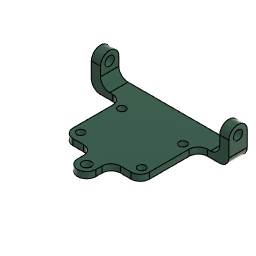
Car_Frame (Autodesk Fusion 360 archive; units mm, degrees)
design "Camera Mount v2"
Autodesk Fusion 360 part; units mm, degrees
sketch "Sketch1" plane through (0, 0, 0) normal (0, 0, 1) x (1, 0, 0)
  line L0 (12.5, 12.5) -> (-12.5, 12.5)
  line L1 (-12.5, 12.5) -> (-12.5, -12.5)
  line L2 (-12.5, -12.5) -> (12.5, -12.5)
  line L3 (12.5, -12.5) -> (12.5, 12.5)
  line L4 (12.5, 12.5) -> (-12.5, -12.5) construction
  line L5 (-12.5, 12.5) -> (12.5, -12.5) construction
  line L6 (10, 4) -> (-10, 4) construction
  line L7 (-10, 4) -> (-10, -9.5) construction
  line L8 (-10, -9.5) -> (10, -9.5) construction
  line L9 (10, -9.5) -> (10, 4) construction
  line L10 (10, 4) -> (-10, -9.5) construction
  line L11 (-10, 4) -> (10, -9.5) construction
  line L12 (0, 0) -> (0, -2.75) construction
  circle A0 centre (-10, -9.5) radius 1.25
  circle A1 centre (-10, 4) radius 1.25
  circle A2 centre (10, 4) radius 1.25
  circle A3 centre (10, -9.5) radius 1.25
  line L13 (-22.5, 12.5) -> (22.5, 12.5)
  line L14 (22.5, 12.5) -> (22.5, 6.5)
  line L15 (22.5, 6.5) -> (-22.5, 6.5)
  line L16 (-22.5, 6.5) -> (-22.5, 12.5)
  line L17 (-12.5, 0) -> (12.5, 0) construction
  line L18 (-22.5, -6.5) -> (-22.5, -12.5) construction
  line L19 (-22.5, -12.5) -> (22.5, -12.5) construction
  line L20 (22.5, -6.5) -> (-22.5, -6.5) construction
  line L21 (22.5, -12.5) -> (22.5, -6.5) construction
  circle A4 centre (0, -17.5) radius 1.5
  line L22 (-3, -17.5) -> (-3, -12.5)
  line L23 (3, -17.5) -> (3, -12.5)
  arc A5 (-3, -17.5) -> (3, -17.5) centre (0, -17.5) ccw
  point P0 (0, -2.75)
  dimension "d1" = 25
  dimension "d2" = 25
  dimension "d3" = 13.5
  dimension "d4" = 20
  dimension "d5" = 3
  dimension "d6" = 2.5
  dimension "d7" = 2.5
  dimension "d8" = 2.5
  dimension "d9" = 2.5
  dimension "d12" = 45
  dimension "d13" = 6
  dimension "d24" = 3
  dimension "d25" = 6
  dimension "d26" = 5
  constraint horizontal L0
  constraint perpendicular L0 L1
  constraint parallel L0 L2
  constraint parallel L1 L3
  constraint coincident L4 L12.start
  constraint coincident L5 L12.start
  constraint coincident L12.start origin
  constraint horizontal L6
  constraint perpendicular L6 L7
  constraint parallel L6 L8
  constraint parallel L7 L9
  constraint coincident L10 P0
  constraint coincident L11 P0
  constraint coincident P0 L12.end
  constraint vertical L12
  constraint coincident L7.end L8.start
  constraint coincident L6.end L7.start
  constraint coincident L6.start L9.end
  constraint coincident L8.end L9.start
  constraint horizontal L13
  constraint vertical L14
  constraint horizontal L15
  constraint vertical L16
  constraint collinear L0 L13
  constraint symmetric L12 L14 L16
  constraint midpoint L1 L17.start
  constraint midpoint L3 L17.end
  constraint symmetric L13.start L17 L18.end
  constraint symmetric L13.end L17 L19.end
  constraint symmetric L14.end L17 L20.start
  constraint symmetric L15.end L17 L18.start
  constraint concentric A4 A5
  constraint coincident L2 L22.end
  constraint coincident L2 L23.end
  constraint vertical L23
  constraint vertical L22
  constraint tangent L22 A5
  constraint tangent L23 A5
  constraint coincident L12 A4.centre
  measures "d1" distance of L1.end L2.end
  measures "d2" distance of L0.end L1.end
  measures "d3" distance of L6.end L7.end
  measures "d4" distance of L6.start L6.end
  measures "d5" distance of L2 L8
  measures "d6" diameter of A0
  measures "d7" diameter of A1
  measures "d8" diameter of A2
  measures "d9" diameter of A3
  measures "d12" distance of L13.start L13.end
  measures "d13" distance of L13.end L14.end
  measures "d24" diameter of A4
  measures "d25" diameter of A5
  measures "d26" distance of L2 A4.centre
extrude "Extrude1" add sketch "Sketch1" along normal blind 2
sketch "Sketch2" plane through (0, 0, 0) normal (1, 0, 0) x (0, 1, 0)
  line L0 (12.5, 0) -> (6.5, 0)
  line L1 (6.5, 0) -> (6.5, 2)
  line L2 (6.5, 2) -> (12.5, 2)
  line L3 (12.5, 2) -> (12.5, 0)
  line L4 (9.5, 2) -> (9.5, 8) construction
  circle A0 centre (9.5, 8) radius 1.5
  circle A1 centre (9.5, 8) radius 3
  line L5 (12.5, 2) -> (12.5, 8)
  line L6 (6.5, 2) -> (6.5, 8)
  dimension "d15" = 3
  dimension "d16" = 6
  dimension "d17" = 6
  constraint midpoint L2 L4.start
  constraint perpendicular L2 L4
  constraint coincident L4.end A0.centre
  constraint concentric A0 A1
  constraint coincident L2.end L3.start
  constraint coincident A1 L5.end
  constraint tangent A1 L5
  constraint coincident L1.end L2.start
  constraint coincident A1 L6.end
  constraint tangent A1 L6
  constraint vertical L6
  constraint vertical L5
  measures "d15" diameter of A0
  measures "d16" diameter of A1
  measures "d17" distance of L4.start L4.end
extrude "Extrude2" add sketch "Sketch2" along normal blind 3 from surface at -22.5 contours L2 A1 L5 L6 | A1
extrude "Extrude3" add sketch "Sketch2" against normal blind 3 from surface at 22.5 contours L2 A1 L5 L6 | A1
fillet "Fillet1" radius 3 10 edges at (12.5, 6.5, 1) (-12.5, 6.5, 1) (-12.5, -12.5, 1) (12.5, -12.5, 1) (-22.5, 9.5, 0) (22.5, 9.5, 0) (-19.5, 9.5, 2) (19.5, 9.5, 2) (3, -12.5, 1) (-3, -12.5, 1)

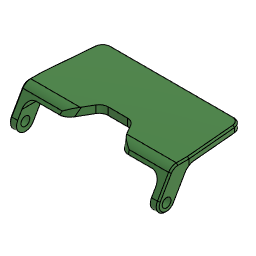
design "Camera Protector"
Autodesk Fusion 360 part; units mm, degrees
sketch "Sketch1" plane through (0, 0, 0) normal (1, 0, 0) x (0, 1, 0)
  circle A0 centre (0, 0) radius 1.5
  line L0 (-2.598076, 1.5) -> (2.020726, 9.5)
  line L1 (2.020726, 9.5) -> (27.020726, 9.5)
  line L2 (27.020726, 9.5) -> (27.020726, 7)
  line L3 (27.020726, 7) -> (7.505553, 7)
  line L4 (7.505553, 7) -> (2.598076, -1.5)
  arc A1 (-2.598076, 1.5) -> (2.598076, -1.5) centre (0, 0) ccw
  line L5 (7.505553, 7) -> (0.57735, 7)
  dimension "d2" = 3
  dimension "d4" = 3
  dimension "d5" = 25
  dimension "d6" = 2.5
  dimension "d7" = 120
  dimension "d8" = 7
  constraint coincident A0.centre A1.centre
  constraint concentric A0 A1
  constraint tangent L0 A1
  constraint horizontal L1
  constraint perpendicular L1 L2
  constraint perpendicular L2 L3
  constraint tangent L4 A1
  constraint parallel L0 L4
  constraint parallel L3 L5
  measures "d2" diameter of A0
  measures "d4" radius of A1
  measures "d7" angle of L0 L1
  measures "d8" distance of A0.centre L3
extrude "Extrude1" add sketch "Sketch1" along normal mid plane 50 contours L0 L1 L2 L3 L5 picked at (12.182335, 8.666667)
extrude "Extrude2" add sketch "Sketch1" against normal blind 2.5 from surface at 25 contours L0 L4 A1 L5 picked at (3.060827, 5.006753)
mirror "Mirror1" about plane through (0, 0, 0) normal (1, 0, 0) of "Extrude2"
sketch "Sketch2" plane through (0, 0, 7) normal (0, 0, -1) x (1, 0, 0)
  line L0 (-22.5, -0.57735) -> (-22.5, -7.505553)
  line L1 (-22.5, -7.505553) -> (-25, -7.505553)
  line L2 (-25, -7.505553) -> (-25, -27.020726)
  line L3 (-25, -27.020726) -> (25, -27.020726)
  line L4 (25, -27.020726) -> (25, -7.505553)
  line L5 (25, -7.505553) -> (22.5, -7.505553)
  line L6 (22.5, -7.505553) -> (22.5, -0.57735)
  line L7 (22.5, -0.57735) -> (-22.5, -0.57735)
  line L8 (-9.618802, -0.57735) -> (-5, -8.57735)
  line L9 (-5, -8.57735) -> (5, -8.57735)
  line L10 (5, -8.57735) -> (9.618802, -0.57735)
  line L11 (0, 0) -> (0, -8.57735) construction
  line L12 (-25, -7.505553) -> (-23.292644, -27.020726)
  line L13 (25, -7.505553) -> (23.292644, -27.020726)
  dimension "d17" = 8
  dimension "d18" = 120
  dimension "d19" = 10
  dimension "d22" = 5
  constraint parallel L7 L9
  constraint coincident L11.start origin
  constraint vertical L11
  constraint symmetric L8 L10 L11
  measures "d17" distance of L7 L9
  measures "d18" angle of L9 L10
  measures "d22" angle of L2 L12
extrude "Extrude3" cut sketch "Sketch2" against normal up to surface (2.5 mm away) contours L7 L8 L9 L10 | L2 L3 L12 | L3 L4 L13 picked at (-1.666667, -3.244017) picked at (-24.430881, -20.515668) picked at (24.430881, -20.515668)
fillet "Fillet1" radius 3 12 edges at (16.892734, 2.020726, 9.5) (-16.892734, 2.020726, 9.5) (23.75, 7.505553, 7) (-23.75, 7.505553, 7) (-5, 8.57735, 8.25) (5, 8.57735, 8.25) (-23.292644, 27.020726, 8.25) (23.292644, 27.020726, 8.25) (22.5, 4.041452, 7) (-22.5, 4.041452, 7) (-9.202135, 1.299038, 8.25) (9.202135, 1.299038, 8.25)
chamfer "Chamfer1" distance 0.5 angle 45 24 edges at (24.266117, 15.893873, 9.5) (22.570421, 26.232558, 9.5) (0, 27.020726, 9.5) (-22.570421, 26.232558, 9.5) (-24.266117, 15.893873, 9.5) (-24.927968, 8.328888, 6.859062) (-24.19035, 16.759899, 7) (-22.570421, 26.232558, 7) (0, 27.020726, 7) (22.570421, 26.232558, 7) (24.19035, 16.759899, 7) (24.927968, 8.328888, 6.859062) (-25, 7.021102, 6.021662) (-25, 4.618802, 2) (-25, -1.5, -2.598076) (-25, -0.721688, 4.75) (-25, 2.252777, 9.098076) (-25, 5.629165, 9.5) (25, 5.629165, 9.5) (25, 2.252777, 9.098076) (25, -0.721688, 4.75) (25, -1.5, -2.598076) (25, 4.618802, 2) (25, 7.021102, 6.021662)
equation "d9 = 45 mm + 5 mm"
